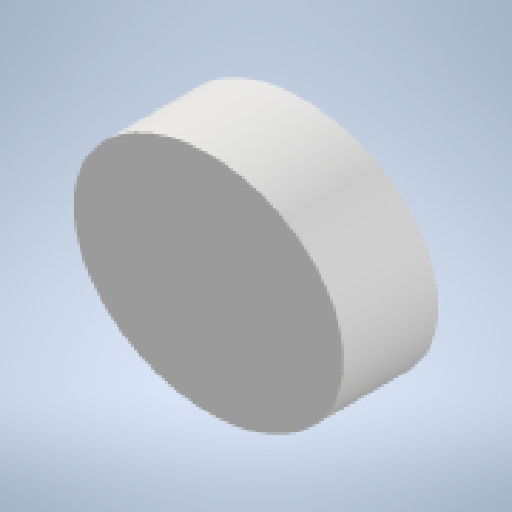
# Autodesk Inventor part: RightCheekPeach
Saved by Autodesk Inventor 2023 (Build 270158000, 158)
## iProperties
Created: 2022-11-09
Part Number: RightCheekPeach
Material: Generic
Document SubType Name: Modeling
Designer: reide
Density: 1 g/cm^3
Appearance: Default
Author: reide
Autodesk Inventor part; units mm, degrees
ref_plane "YZ Plane" through (0, 0, 0) normal (1, 0, 0) x (0, 1, 0)
ref_plane "XZ Plane" through (0, 0, 0) normal (0, 1, 0) x (-1, 0, 0)
ref_plane "XY Plane" through (0, 0, 0) normal (0, 0, 1) x (1, 0, 0)
sketch "Sketch1" plane through (0, 0, 0) normal (0, 0, 1) x (1, 0, 0)
  ellipse E0 centre (0, 0) end of major axis (-3, 0) minor radius 2.4928 projected
  ellipse E1 centre (0, 0) end of major axis (2.85, 0) minor radius 2.3682
  constraints: 1 centre point, 1 coincident, 2 other
extrude "Extrusion1" add sketch "Sketch1" along normal blind 2 contours E1
body "Solid1"
